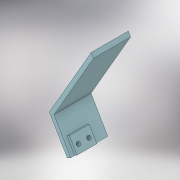
# Autodesk Inventor part: TA09
Saved by Autodesk Inventor 2017 (Build 210142000, 142)
## iProperties
Created: 2019-04-11
Part Number: TA09
Material: ABS Plastic
Document SubType Name: Modeling
Designer: Dell
Density: 1.06 g/cm^3
Appearance: Sky Blue Dark(3)
Author: Dell
Autodesk Inventor part; units mm, degrees
ref_plane "YZ Plane" through (0, 0, 0) normal (1, 0, 0) x (0, 1, 0)
ref_plane "XZ Plane" through (0, 0, 0) normal (0, 1, 0) x (-1, 0, 0)
ref_plane "XY Plane" through (0, 0, 0) normal (0, 0, 1) x (1, 0, 0)
sketch "Sketch1" plane through (0, 0, 0) normal (0, 0, 1) x (1, 0, 0)
  line L0 (57.5, 0) -> (28.75, -49.7965) construction
  line L1 (28.75, -49.7965) -> (-28.75, -49.7965) construction
  line L2 (-28.75, -49.7965) -> (-57.5, 0) construction
  line L3 (-57.5, 0) -> (-28.75, 49.7965) construction
  line L4 (-28.75, 49.7965) -> (28.75, 49.7965) construction
  line L5 (28.75, 49.7965) -> (57.5, 0) construction
  line L6 (-31.6368, 54.7965) -> (-63.2735, 0) construction
  line L7 (-63.2735, 0) -> (-31.6368, -54.7965) construction
  line L8 (-31.6368, -54.7965) -> (31.6368, -54.7965) construction
  line L9 (31.6368, -54.7965) -> (63.2735, 0) construction
  line L10 (63.2735, 0) -> (31.6368, 54.7965) construction
  line L11 (31.6368, 54.7965) -> (-31.6368, 54.7965) construction
  line L12 (-47.9466, -16.547) -> (-52.2767, -19.047) construction
  line L13 (-45.4466, -20.8771) -> (-49.7767, -23.3771)
  line L14 (-45.4466, -20.8771) -> (-57.5, 0)
  line L15 (-49.7767, -23.3771) -> (-63.2735, 0)
  line L16 (-63.2735, 0) -> (-31.6368, 54.7965)
  line L17 (-31.6368, 54.7965) -> (-28.75, 49.7965)
  line L18 (-28.75, 49.7965) -> (-57.5, 0)
  point P0 (0, 0)
  point P1 (0, 0)
  dimension "d0" = 115
  dimension "d1" = 5
  dimension "d2" = 19.1068
  dimension "d3" = 5
  constraints: 38 end point, 4 point on line, 3 collinear, 2 perpendicular, 1 coincident, 1 horizontal alignment, 18 other
  measures "d0" distance of L2.end L0.start
  measures "d1" distance between parallel lines of L3 L6
  measures "d2" distance from line of L2.end L12
  measures "d3" distance between parallel lines of L12 L13
extrude "Extrusion1" add sketch "Sketch1" along normal blind 35
sketch "Sketch2" plane through (-57.5, 0, 35) normal (0.8660254, 0.5, 0) x (0, 0, -1)
  circle A0 centre (17.5, -19.1068) radius 1.5 construction
  line L0 (35, -24.1068) -> (0, -24.1068) projected
  line L1 (21.5, -19.1068) -> (13.5, -19.1068) construction
  circle A1 centre (21.5, -19.1068) radius 1.5
  circle A2 centre (13.5, -19.1068) radius 1.5
  point P0 (35, -28.75)
  point P1 (17.5, -24.1068)
  dimension "d6" = 3
  dimension "d7" = 5
  dimension "d14" = 8
  dimension "d15" = 3
  dimension "d16" = 3
  constraints: 3 centre point, 3 coincident, 2 end point, 2 midpoint, 1 horizontal, 1 vertical alignment
  measures "d6" diameter of A0
  measures "d7" distance from line of L0 A0.centre
  measures "d14" distance of L1.start L1.end
  measures "d15" diameter of A1
  measures "d16" diameter of A2
extrude "Extrusion2" cut sketch "Sketch2" against normal through all
sketch "Sketch3" plane through (0, 0, 35) normal (0, 0, 1) x (1, 0, 0)
  line L0 (-45.4466, -20.8771) -> (-57.5, 0) construction
  line L1 (-57.5, 0) -> (-28.75, 49.7965) construction
  line L2 (-30.4821, 50.7965) -> (-59.8094, 0) construction
  line L3 (-59.8094, 0) -> (-47.1786, -21.8771) construction
  line L4 (-51.5267, -20.346) -> (-53.0267, -17.7479) construction
  line L5 (-48.6966, -15.2479) -> (-47.1966, -17.846) construction
  line L6 (-51.1966, -10.9178) -> (-52.9286, -11.9178)
  line L7 (-51.1966, -10.9178) -> (-57.5, 0)
  line L8 (-57.5, 0) -> (-28.75, 49.7965)
  line L9 (-28.75, 49.7965) -> (-29.9047, 51.7965)
  line L10 (-28.75, 49.7965) -> (-31.6368, 54.7965) projected
  line L11 (-29.9047, 51.7965) -> (-59.8094, 0)
  line L12 (-59.8094, 0) -> (-52.9286, -11.9178)
  line L13 (-49.7767, -23.3771) -> (-45.4466, -20.8771) projected
  point P0 (0, 0)
  dimension "d10" = 2
  dimension "d17" = 11.5
  constraints: 16 end point, 4 point on line, 2 collinear, 1 parallel, 1 perpendicular, 1 other
  measures "d10" distance between parallel lines of L1 L2
  measures "d17" distance between parallel lines of L13 L6
extrude "Extrusion3" cut sketch "Sketch3" against normal through all
sketch "Sketch4" plane through (-45.4466, -20.8771, 35) normal (0.8660254, 0.5, 0) x (0, 0, -1)
  line L0 (35, 0) -> (0, 0) construction
  line L1 (35, 11.5) -> (0, 11.5) construction
  line L2 (10, 0) -> (25, 0)
  line L3 (25, 0) -> (25, 11.5)
  line L4 (25, 11.5) -> (10, 11.5)
  line L5 (10, 11.5) -> (10, 0)
  circle A0 centre (13.5, 5) radius 1.5 construction
  line L6 (13.5, 5) -> (21.5, 5) construction
  circle A1 centre (21.5, 5) radius 1.5 construction
  line L7 (10, 11.5) -> (0, 11.5)
  line L8 (0, 11.5) -> (0, 0)
  line L9 (0, 0) -> (10, 0)
  line L10 (10, 0) -> (10, 11.5)
  line L11 (35, 11.5) -> (35, 0) projected
  line L12 (25, 11.5) -> (35, 11.5)
  line L13 (35, 11.5) -> (35, 0)
  line L14 (35, 0) -> (25, 0)
  line L15 (25, 0) -> (25, 11.5)
  point P0 (35, -4.6432)
  point P1 (17.5, 5)
  point P2 (17.5, 11.5)
  point P3 (17.5, 11.5)
  dimension "d18" = 15
  constraints: 26 end point, 6 parallel, 4 horizontal, 3 midpoint, 3 perpendicular, 2 point on line, 2 vertical alignment, 1 coincident
  measures "d18" distance between parallel lines of L5 L3
extrude "Extrusion4" cut sketch "Sketch4" against normal blind 2 contours L9 L8 L7 L5 | L3 L12 L11 L14
sketch "Sketch5" plane through (-49.7767, -23.3771, 0) normal (-0.8660254, -0.5, 0) x (0, 0, 1)
  line L0 (0, 0) -> (35, 0) projected
  line L1 (0, 58.6303) -> (35, 58.6303) projected
  line L2 (35, 0) -> (28, 0)
  line L3 (28, 0) -> (28, 58.6303)
  line L4 (28, 58.6303) -> (35, 58.6303)
  line L5 (35, 58.6303) -> (35, 0)
  point P0 (0, -4.6432)
  dimension "d21" = 7
  constraints: 8 end point, 2 parallel, 1 horizontal, 1 perpendicular, 1 point on line
  measures "d21" distance between parallel lines of L5 L3
extrude "Extrusion5" cut sketch "Sketch5" against normal through all
body "Solid1"
